Autodesk Fusion 360 part; units mm, degrees
(part 5 of 7)
  line L374 (70.3431, -42.6334) -> (70.3628, -42.5576)
  line L375 (70.3628, -42.5576) -> (70.3811, -42.4808)
  line L376 (70.3811, -42.4808) -> (70.2693, -42.3959)
  line L377 (70.2693, -42.3959) -> (70.1562, -42.3126)
  line L378 (70.1562, -42.3126) -> (70.0419, -42.2311)
  line L379 (70.0419, -42.2311) -> (69.974, -42.2713)
  line L380 (69.974, -42.2713) -> (69.9075, -42.3127)
  line L381 (69.9075, -42.3127) -> (69.8424, -42.3551)
  line L382 (69.8424, -42.3551) -> (69.7789, -42.3987)
  line L383 (69.7789, -42.3987) -> (69.7169, -42.4435)
  line L384 (69.7169, -42.4435) -> (69.6565, -42.4895)
  line L385 (69.6565, -42.4895) -> (69.5979, -42.5367)
  line L386 (69.5979, -42.5367) -> (69.5413, -42.5853)
  line L387 (69.5413, -42.5853) -> (69.4867, -42.6354)
  line L388 (69.4867, -42.6354) -> (69.4346, -42.6871)
  line L389 (69.4346, -42.6871) -> (69.3854, -42.7407)
  line L390 (69.3854, -42.7407) -> (69.3406, -42.7973)
  line L391 (69.3406, -42.7973) -> (69.0945, -43.1707)
  line L392 (69.0945, -43.1707) -> (68.9167, -43.0569)
  line L393 (68.9167, -43.0569) -> (68.7359, -42.9478)
  line L394 (68.7359, -42.9478) -> (68.5524, -42.8434)
  line L395 (68.5524, -42.8434) -> (68.3661, -42.744)
  line L396 (68.3661, -42.744) -> (68.5716, -42.3467)
  line L397 (68.5716, -42.3467) -> (68.599, -42.28)
  line L398 (68.599, -42.28) -> (68.6218, -42.2108)
  line L399 (68.6218, -42.2108) -> (68.6414, -42.1401)
  line L400 (68.6414, -42.1401) -> (68.6584, -42.068)
  line L401 (68.6584, -42.068) -> (68.6731, -41.9948)
  line L402 (68.6731, -41.9948) -> (68.6857, -41.9206)
  line L403 (68.6857, -41.9206) -> (68.6963, -41.8455)
  line L404 (68.6963, -41.8455) -> (68.705, -41.7695)
  line L405 (68.705, -41.7695) -> (68.712, -41.6928)
  line L406 (68.712, -41.6928) -> (68.7172, -41.6152)
  line L407 (68.7172, -41.6152) -> (68.7208, -41.537)
  line L408 (68.7208, -41.537) -> (68.7227, -41.4581)
  line L409 (68.7227, -41.4581) -> (68.5957, -41.3983)
  line L410 (68.5957, -41.3983) -> (68.4678, -41.3403)
  line L411 (68.4678, -41.3403) -> (68.339, -41.2843)
  line L412 (68.339, -41.2843) -> (68.2809, -41.3378)
  line L413 (68.2809, -41.3378) -> (68.2245, -41.3921)
  line L414 (68.2245, -41.3921) -> (68.1697, -41.4471)
  line L415 (68.1697, -41.4471) -> (68.1165, -41.503)
  line L416 (68.1165, -41.503) -> (68.0652, -41.5597)
  line L417 (68.0652, -41.5597) -> (68.0157, -41.6172)
  line L418 (68.0157, -41.6172) -> (67.9683, -41.6756)
  line L419 (67.9683, -41.6756) -> (67.923, -41.7349)
  line L420 (67.923, -41.7349) -> (67.88, -41.7952)
  line L421 (67.88, -41.7952) -> (67.8398, -41.8566)
  line L422 (67.8398, -41.8566) -> (67.8028, -41.9193)
  line L423 (67.8028, -41.9193) -> (67.7707, -41.984)
  line L424 (67.7707, -41.984) -> (67.6076, -42.4004)
  line L425 (67.6076, -42.4004) -> (67.41, -42.326)
  line L426 (67.41, -42.326) -> (67.2106, -42.2569)
  line L427 (67.2106, -42.2569) -> (67.0093, -42.193)
  line L428 (67.0093, -42.193) -> (66.8065, -42.1344)
  line L429 (66.8065, -42.1344) -> (66.9248, -41.7032)
  line L430 (66.9248, -41.7032) -> (66.9378, -41.6322)
  line L431 (66.9378, -41.6322) -> (66.9457, -41.5598)
  line L432 (66.9457, -41.5598) -> (66.9502, -41.4865)
  line L433 (66.9502, -41.4865) -> (66.9518, -41.4125)
  line L434 (66.9518, -41.4125) -> (66.951, -41.3378)
  line L435 (66.951, -41.3378) -> (66.9479, -41.2627)
  line L436 (66.9479, -41.2627) -> (66.9426, -41.187)
  line L437 (66.9426, -41.187) -> (66.9354, -41.1108)
  line L438 (66.9354, -41.1108) -> (66.9262, -41.0343)
  line L439 (66.9262, -41.0343) -> (66.9152, -40.9574)
  line L440 (66.9152, -40.9574) -> (66.9024, -40.8801)
  line L441 (66.9024, -40.8801) -> (66.8879, -40.8025)
  line L442 (66.8879, -40.8025) -> (66.7512, -40.7704)
  line L443 (66.7512, -40.7704) -> (66.614, -40.7403)
  line L444 (66.614, -40.7403) -> (66.4764, -40.7123)
  line L445 (66.4764, -40.7123) -> (66.4308, -40.7767)
  line L446 (66.4308, -40.7767) -> (66.3868, -40.8415)
  line L447 (66.3868, -40.8415) -> (66.3447, -40.9068)
  line L448 (66.3447, -40.9068) -> (66.3043, -40.9725)
  line L449 (66.3043, -40.9725) -> (66.2659, -41.0386)
  line L450 (66.2659, -41.0386) -> (66.2295, -41.1051)
  line L451 (66.2295, -41.1051) -> (66.1952, -41.1721)
  line L452 (66.1952, -41.1721) -> (66.1632, -41.2396)
  line L453 (66.1632, -41.2396) -> (66.1337, -41.3075)
  line L454 (66.1337, -41.3075) -> (66.1071, -41.3759)
  line L455 (66.1071, -41.3759) -> (66.084, -41.4449)
  line L456 (66.084, -41.4449) -> (66.066, -41.5149)
  line L457 (66.066, -41.5149) -> (65.9931, -41.9561)
  line L458 (65.9931, -41.9561) -> (65.7844, -41.9244)
  line L459 (65.7844, -41.9244) -> (65.5749, -41.8982)
  line L460 (65.5749, -41.8982) -> (65.3648, -41.8776)
  line L461 (65.3648, -41.8776) -> (65.1542, -41.8625)
  line L462 (65.1542, -41.8625) -> (65.1803, -41.416)
  line L463 (65.1803, -41.416) -> (65.1782, -41.3439)
  line L464 (65.1782, -41.3439) -> (65.1709, -41.2714)
  line L465 (65.1709, -41.2714) -> (65.16, -41.1988)
  line L466 (65.16, -41.1988) -> (65.1462, -41.1261)
  line L467 (65.1462, -41.1261) -> (65.1299, -41.0533)
  line L468 (65.1299, -41.0533) -> (65.1112, -40.9804)
  line L469 (65.1112, -40.9804) -> (65.0903, -40.9074)
  line L470 (65.0903, -40.9074) -> (65.0674, -40.8345)
  line L471 (65.0674, -40.8345) -> (65.0425, -40.7615)
  line L472 (65.0425, -40.7615) -> (65.0158, -40.6885)
  line L473 (65.0158, -40.6885) -> (64.9872, -40.6156)
  line L474 (64.9872, -40.6156) -> (64.9569, -40.5428)
  line L475 (64.9569, -40.5428) -> (64.8165, -40.5397)
  line L476 (64.8165, -40.5397) -> (64.6761, -40.5388)
  line L477 (64.6761, -40.5388) -> (64.5356, -40.5401)
  line L478 (64.5356, -40.5401) -> (64.5044, -40.6125)
  line L479 (64.5044, -40.6125) -> (64.4749, -40.6851)
  line L480 (64.4749, -40.6851) -> (64.4472, -40.7577)
  line L481 (64.4472, -40.7577) -> (64.4214, -40.8303)
  line L482 (64.4214, -40.8303) -> (64.3975, -40.903)
  line L483 (64.3975, -40.903) -> (64.3758, -40.9757)
  line L484 (64.3758, -40.9757) -> (64.3561, -41.0483)
  line L485 (64.3561, -41.0483) -> (64.3389, -41.1209)
  line L486 (64.3389, -41.1209) -> (64.3242, -41.1935)
  line L487 (64.3242, -41.1935) -> (64.3124, -41.2659)
  line L488 (64.3124, -41.2659) -> (64.3041, -41.3383)
  line L489 (64.3041, -41.3383) -> (64.3011, -41.4104)
  line L490 (64.3011, -41.4104) -> (64.3215, -41.8572)
  line L491 (64.3215, -41.8572) -> (64.1107, -41.8696)
  line L492 (64.1107, -41.8696) -> (63.9004, -41.8875)
  line L493 (63.9004, -41.8875) -> (63.6905, -41.911)
  line L494 (63.6905, -41.911) -> (63.4814, -41.94)
  line L495 (63.4814, -41.94) -> (63.4141, -41.4979)
  line L496 (63.4141, -41.4979) -> (63.3971, -41.4277)
  line L497 (63.3971, -41.4277) -> (63.3749, -41.3584)
  line L498 (63.3749, -41.3584) -> (63.3491, -41.2897)
  line L499 (63.3491, -41.2897) -> (63.3205, -41.2214)
  line L500 (63.3205, -41.2214) -> (63.2894, -41.1535)
  line L501 (63.2894, -41.1535) -> (63.256, -41.0861)
  line L502 (63.256, -41.0861) -> (63.2204, -41.0191)
  line L503 (63.2204, -41.0191) -> (63.1828, -40.9525)
  line L504 (63.1828, -40.9525) -> (63.1433, -40.8863)
  line L505 (63.1433, -40.8863) -> (63.102, -40.8205)
  line L506 (63.102, -40.8205) -> (63.0589, -40.7551)
  line L507 (63.0589, -40.7551) -> (63.0141, -40.6901)
  line L508 (63.0141, -40.6901) -> (62.8761, -40.7164)
  line L509 (62.8761, -40.7164) -> (62.7386, -40.7447)
  line L510 (62.7386, -40.7447) -> (62.6015, -40.7751)
  line L511 (62.6015, -40.7751) -> (62.5859, -40.8525)
  line L512 (62.5859, -40.8525) -> (62.5722, -40.9296)
  line L513 (62.5722, -40.9296) -> (62.5602, -41.0063)
  line L514 (62.5602, -41.0063) -> (62.5501, -41.0827)
  line L515 (62.5501, -41.0827) -> (62.5418, -41.1588)
  line L516 (62.5418, -41.1588) -> (62.5356, -41.2344)
  line L517 (62.5356, -41.2344) -> (62.5315, -41.3095)
  line L518 (62.5315, -41.3095) -> (62.5297, -41.3842)
  line L519 (62.5297, -41.3842) -> (62.5304, -41.4582)
  line L520 (62.5304, -41.4582) -> (62.534, -41.5315)
  line L521 (62.534, -41.5315) -> (62.5409, -41.604)
  line L522 (62.5409, -41.604) -> (62.553, -41.6752)
  line L523 (62.553, -41.6752) -> (62.6658, -42.1079)
  line L524 (62.6658, -42.1079) -> (62.4622, -42.1639)
  line L525 (62.4622, -42.1639) -> (62.2602, -42.2252)
  line L526 (62.2602, -42.2252) -> (62.0599, -42.2918)
  line L527 (62.0599, -42.2918) -> (61.8613, -42.3636)
  line L528 (61.8613, -42.3636) -> (61.7036, -41.9451)
  line L529 (61.7036, -41.9451) -> (61.6724, -41.8801)
  line L530 (61.6724, -41.8801) -> (61.6362, -41.8169)
  line L531 (61.6362, -41.8169) -> (61.5967, -41.755)
  line L532 (61.5967, -41.755) -> (61.5546, -41.6941)
  line L533 (61.5546, -41.6941) -> (61.51, -41.6342)
  line L534 (61.51, -41.6342) -> (61.4633, -41.5752)
  line L535 (61.4633, -41.5752) -> (61.4146, -41.5171)
  line L536 (61.4146, -41.5171) -> (61.3639, -41.4598)
  line L537 (61.3639, -41.4598) -> (61.3115, -41.4032)
  line L538 (61.3115, -41.4032) -> (61.2574, -41.3474)
  line L539 (61.2574, -41.3474) -> (61.2017, -41.2925)
  line L540 (61.2017, -41.2925) -> (61.1443, -41.2382)
  line L541 (61.1443, -41.2382) -> (61.0148, -41.2926)
  line L542 (61.0148, -41.2926) -> (60.8862, -41.3489)
  line L543 (60.8862, -41.3489) -> (60.7584, -41.4071)
  line L544 (60.7584, -41.4071) -> (60.7593, -41.486)
  line L545 (60.7593, -41.486) -> (60.7619, -41.5643)
  line L546 (60.7619, -41.5643) -> (60.7661, -41.6419)
  line L547 (60.7661, -41.6419) -> (60.7721, -41.7187)
  line L548 (60.7721, -41.7187) -> (60.7799, -41.7948)
  line L549 (60.7799, -41.7948) -> (60.7895, -41.8701)
  line L550 (60.7895, -41.8701) -> (60.8011, -41.9444)
  line L551 (60.8011, -41.9444) -> (60.8149, -42.0178)
  line L552 (60.8149, -42.0178) -> (60.831, -42.0901)
  line L553 (60.831, -42.0901) -> (60.8497, -42.1611)
  line L554 (60.8497, -42.1611) -> (60.8715, -42.2305)
  line L555 (60.8715, -42.2305) -> (60.8981, -42.2976)
  line L556 (60.8981, -42.2976) -> (61.0985, -42.6974)
  line L557 (61.0985, -42.6974) -> (60.911, -42.7945)
  line L558 (60.911, -42.7945) -> (60.7261, -42.8965)
  line L559 (60.7261, -42.8965) -> (60.544, -43.0033)
  line L560 (60.544, -43.0033) -> (60.3647, -43.1148)
  line L561 (60.3647, -43.1148) -> (60.1234, -42.7383)
  line L562 (60.1234, -42.7383) -> (60.0794, -42.6811)
  line L563 (60.0794, -42.6811) -> (60.0308, -42.6268)
  line L564 (60.0308, -42.6268) -> (59.9794, -42.5745)
  line L565 (59.9794, -42.5745) -> (59.9255, -42.5237)
  line L566 (59.9255, -42.5237) -> (59.8694, -42.4744)
  line L567 (59.8694, -42.4744) -> (59.8115, -42.4264)
  line L568 (59.8115, -42.4264) -> (59.7517, -42.3797)
  line L569 (59.7517, -42.3797) -> (59.6903, -42.3341)
  line L570 (59.6903, -42.3341) -> (59.6273, -42.2897)
  line L571 (59.6273, -42.2897) -> (59.5628, -42.2464)
  line L572 (59.5628, -42.2464) -> (59.4968, -42.2042)
  line L573 (59.4968, -42.2042) -> (59.4294, -42.1631)
  line L574 (59.4294, -42.1631) -> (59.3141, -42.2432)
  line L575 (59.3141, -42.2432) -> (59.1999, -42.325)
  line L576 (59.1999, -42.325) -> (59.087, -42.4085)
  line L577 (59.087, -42.4085) -> (59.1043, -42.4855)
  line L578 (59.1043, -42.4855) -> (59.1231, -42.5615)
  line L579 (59.1231, -42.5615) -> (59.1434, -42.6365)
  line L580 (59.1434, -42.6365) -> (59.1652, -42.7105)
  line L581 (59.1652, -42.7105) -> (59.1886, -42.7833)
  line L582 (59.1886, -42.7833) -> (59.2137, -42.8549)
  line L583 (59.2137, -42.8549) -> (59.2405, -42.9252)
  line L584 (59.2405, -42.9252) -> (59.2693, -42.9941)
  line L585 (59.2693, -42.9941) -> (59.3, -43.0614)
  line L586 (59.3, -43.0614) -> (59.3331, -43.127)
  line L587 (59.3331, -43.127) -> (59.3689, -43.1904)
  line L588 (59.3689, -43.1904) -> (59.4088, -43.2505)
  line L589 (59.4088, -43.2505) -> (59.6879, -43.5999)
  line L590 (59.6879, -43.5999) -> (59.5247, -43.7339)
  line L591 (59.5247, -43.7339) -> (59.3651, -43.872)
  line L592 (59.3651, -43.872) -> (59.2092, -44.0144)
  line L593 (59.2092, -44.0144) -> (59.057, -44.1608)
  line L594 (59.057, -44.1608) -> (58.7427, -43.8426)
  line L595 (58.7427, -43.8426) -> (58.6877, -43.7959)
  line L596 (58.6877, -43.7959) -> (58.629, -43.7529)
  line L597 (58.629, -43.7529) -> (58.5677, -43.7124)
  line L598 (58.5677, -43.7124) -> (58.5045, -43.6739)
  line L599 (58.5045, -43.6739) -> (58.4394, -43.6373)
  line L600 (58.4394, -43.6373) -> (58.3727, -43.6024)
  line L601 (58.3727, -43.6024) -> (58.3045, -43.5691)
  line L602 (58.3045, -43.5691) -> (58.235, -43.5373)
  line L603 (58.235, -43.5373) -> (58.1641, -43.507)
  line L604 (58.1641, -43.507) -> (58.092, -43.4781)
  line L605 (58.092, -43.4781) -> (58.0187, -43.4505)
  line L606 (58.0187, -43.4505) -> (57.9443, -43.4243)
  line L607 (57.9443, -43.4243) -> (57.8481, -43.5266)
  line L608 (57.8481, -43.5266) -> (57.7534, -43.6304)
  line L609 (57.7534, -43.6304) -> (57.6604, -43.7355)
  line L610 (57.6604, -43.7355) -> (57.6933, -43.8072)
  line L611 (57.6933, -43.8072) -> (57.7275, -43.8777)
  line L612 (57.7275, -43.8777) -> (57.7629, -43.9469)
  line L613 (57.7629, -43.9469) -> (57.7996, -44.0147)
  line L614 (57.7996, -44.0147) -> (57.8377, -44.081)
  line L615 (57.8377, -44.081) -> (57.8771, -44.1458)
  line L616 (57.8771, -44.1458) -> (57.918, -44.209)
  line L617 (57.918, -44.209) -> (57.9604, -44.2704)
  line L618 (57.9604, -44.2704) -> (58.0045, -44.3299)
  line L619 (58.0045, -44.3299) -> (58.0504, -44.3872)
  line L620 (58.0504, -44.3872) -> (58.0986, -44.4417)
  line L621 (58.0986, -44.4417) -> (58.1502, -44.4922)
  line L622 (58.1502, -44.4922) -> (58.4959, -44.776)
  line L623 (58.4959, -44.776) -> (58.3641, -44.9409)
  line L624 (58.3641, -44.9409) -> (58.2367, -45.1093)
  line L625 (58.2367, -45.1093) -> (58.1137, -45.2809)
  line L626 (58.1137, -45.2809) -> (57.9953, -45.4557)
  line L627 (57.9953, -45.4557) -> (57.6217, -45.2099)
  line L628 (57.6217, -45.2099) -> (57.5582, -45.1756)
  line L629 (57.5582, -45.1756) -> (57.4918, -45.1457)
  line L630 (57.4918, -45.1457) -> (57.4235, -45.1189)
  line L631 (57.4235, -45.1189) -> (57.3536, -45.0944)
  line L632 (57.3536, -45.0944) -> (57.2824, -45.0721)
  line L633 (57.2824, -45.0721) -> (57.2099, -45.0519)
  line L634 (57.2099, -45.0519) -> (57.1363, -45.0335)
  line L635 (57.1363, -45.0335) -> (57.0617, -45.0168)
  line L636 (57.0617, -45.0168) -> (56.986, -45.0019)
  line L637 (56.986, -45.0019) -> (56.9095, -44.9886)
  line L638 (56.9095, -44.9886) -> (56.832, -44.9769)
  line L639 (56.832, -44.9769) -> (56.7538, -44.9667)
  line L640 (56.7538, -44.9667) -> (56.681, -45.0868)
  line L641 (56.681, -45.0868) -> (56.61, -45.2079)
  line L642 (56.61, -45.2079) -> (56.5408, -45.3302)
  line L643 (56.5408, -45.3302) -> (56.5879, -45.3935)
  line L644 (56.5879, -45.3935) -> (56.636, -45.4553)
  line L645 (56.636, -45.4553) -> (56.6851, -45.5156)
  line L646 (56.6851, -45.5156) -> (56.7351, -45.5742)
  line L647 (56.7351, -45.5742) -> (56.7861, -45.6312)
  line L648 (56.7861, -45.6312) -> (56.8381, -45.6864)
  line L649 (56.8381, -45.6864) -> (56.8912, -45.7397)
  line L650 (56.8912, -45.7397) -> (56.9455, -45.791)
  line L651 (56.9455, -45.791) -> (57.001, -45.84)
  line L652 (57.001, -45.84) -> (57.0578, -45.8865)
  line L653 (57.0578, -45.8865) -> (57.1163, -45.9298)
  line L654 (57.1163, -45.9298) -> (57.1773, -45.9685)
  line L655 (57.1773, -45.9685) -> (57.5744, -46.1742)
  line L656 (57.5744, -46.1742) -> (57.4797, -46.3629)
  line L657 (57.4797, -46.3629) -> (57.3901, -46.5541)
  line L658 (57.3901, -46.5541) -> (57.3055, -46.7475)
  line L659 (57.3055, -46.7475) -> (57.2261, -46.9431)
  line L660 (57.2261, -46.9431) -> (56.8096, -46.7803)
  line L661 (56.8096, -46.7803) -> (56.7403, -46.76)
  line L662 (56.7403, -46.76) -> (56.6691, -46.7446)
  line L663 (56.6691, -46.7446) -> (56.5967, -46.7325)
  line L664 (56.5967, -46.7325) -> (56.5233, -46.7231)
  line L665 (56.5233, -46.7231) -> (56.449, -46.7162)
  line L666 (56.449, -46.7162) -> (56.3739, -46.7114)
  line L667 (56.3739, -46.7114) -> (56.2981, -46.7087)
  line L668 (56.2981, -46.7087) -> (56.2216, -46.708)
  line L669 (56.2216, -46.708) -> (56.1445, -46.7091)
  line L670 (56.1445, -46.7091) -> (56.0668, -46.712)
  line L671 (56.0668, -46.712) -> (55.9887, -46.7166)
  line L672 (55.9887, -46.7166) -> (55.91, -46.7229)
  line L673 (55.91, -46.7229) -> (55.8637, -46.8555)
  line L674 (55.8637, -46.8555) -> (55.8195, -46.9888)
  line L675 (55.8195, -46.9888) -> (55.7773, -47.1227)
  line L676 (55.7773, -47.1227) -> (55.8365, -47.1749)
  line L677 (55.8365, -47.1749) -> (55.8964, -47.2253)
  line L678 (55.8964, -47.2253) -> (55.9569, -47.2741)
  line L679 (55.9569, -47.2741) -> (56.018, -47.3211)
  line L680 (56.018, -47.3211) -> (56.0797, -47.3662)
  line L681 (56.0797, -47.3662) -> (56.1421, -47.4094)
  line L682 (56.1421, -47.4094) -> (56.2052, -47.4505)
  line L683 (56.2052, -47.4505) -> (56.2689, -47.4894)
  line L684 (56.2689, -47.4894) -> (56.3334, -47.5258)
  line L685 (56.3334, -47.5258) -> (56.3986, -47.5594)
  line L686 (56.3986, -47.5594) -> (56.4649, -47.5896)
  line L687 (56.4649, -47.5896) -> (56.5325, -47.6147)
  line L688 (56.5325, -47.6147) -> (56.9637, -47.7334)
  line L689 (56.9637, -47.7334) -> (56.9104, -47.9377)
  line L690 (56.9104, -47.9377) -> (56.8625, -48.1433)
  line L691 (56.8625, -48.1433) -> (56.82, -48.3501)
  line L692 (56.82, -48.3501) -> (56.7829, -48.558)
  line L693 (56.7829, -48.558) -> (56.3416, -48.4853)
  line L694 (56.3416, -48.4853) -> (56.2697, -48.4798)
  line L695 (56.2697, -48.4798) -> (56.1969, -48.4796)
  line L696 (56.1969, -48.4796) -> (56.1235, -48.4828)
  line L697 (56.1235, -48.4828) -> (56.0497, -48.4889)
  line L698 (56.0497, -48.4889) -> (55.9756, -48.4975)
  line L699 (55.9756, -48.4975) -> (55.9011, -48.5085)
  line L700 (55.9011, -48.5085) -> (55.8264, -48.5216)
  line L701 (55.8264, -48.5216) -> (55.7515, -48.5368)
  line L702 (55.7515, -48.5368) -> (55.6763, -48.5539)
  line L703 (55.6763, -48.5539) -> (55.6009, -48.5729)
  line L704 (55.6009, -48.5729) -> (55.5254, -48.5937)
  line L705 (55.5254, -48.5937) -> (55.4498, -48.6162)
  line L706 (55.4498, -48.6162) -> (55.4321, -48.7555)
  line L707 (55.4321, -48.7555) -> (55.4165, -48.8951)
  line L708 (55.4165, -48.8951) -> (55.4031, -49.0349)
  line L709 (55.4031, -49.0349) -> (55.4719, -49.0735)
  line L710 (55.4719, -49.0735) -> (55.5409, -49.1105)
  line L711 (55.5409, -49.1105) -> (55.6103, -49.1456)
  line L712 (55.6103, -49.1456) -> (55.6798, -49.1788)
  line L713 (55.6798, -49.1788) -> (55.7496, -49.2101)
  line L714 (55.7496, -49.2101) -> (55.8196, -49.2394)
  line L715 (55.8196, -49.2394) -> (55.8898, -49.2665)
  line L716 (55.8898, -49.2665) -> (55.9602, -49.2913)
  line L717 (55.9602, -49.2913) -> (56.0308, -49.3135)
  line L718 (56.0308, -49.3135) -> (56.1017, -49.3328)
  line L719 (56.1017, -49.3328) -> (56.1727, -49.3486)
  line L720 (56.1727, -49.3486) -> (56.2441, -49.3591)
  line L721 (56.2441, -49.3591) -> (56.6906, -49.3855)
  line L722 (56.6906, -49.3855) -> (56.6809, -49.5964)
  line L723 (56.6809, -49.5964) -> (56.6768, -49.8075)
  line L724 (56.6768, -49.8075) -> (56.6782, -50.0186)
  line L725 (56.6782, -50.0186) -> (56.6852, -50.2297)
  line L726 (56.6852, -50.2297) -> (56.2384, -50.2504)
  line L727 (56.2384, -50.2504) -> (56.1669, -50.26)
  line L728 (56.1669, -50.26) -> (56.0956, -50.2748)
  line L729 (56.0956, -50.2748) -> (56.0245, -50.2932)
  line L730 (56.0245, -50.2932) -> (55.9536, -50.3145)
  line L731 (55.9536, -50.3145) -> (55.8829, -50.3384)
  line L732 (55.8829, -50.3384) -> (55.8124, -50.3646)
  line L733 (55.8124, -50.3646) -> (55.742, -50.393)
  line L734 (55.742, -50.393) -> (55.6718, -50.4234)
  line L735 (55.6718, -50.4234) -> (55.6019, -50.4558)
  line L736 (55.6019, -50.4558) -> (55.5321, -50.49)
  line L737 (55.5321, -50.49) -> (55.4626, -50.526)
  line L738 (55.4626, -50.526) -> (55.3933, -50.5638)
  line L739 (55.3933, -50.5638) -> (55.405, -50.7037)
  line L740 (55.405, -50.7037) -> (55.4187, -50.8435)
  line L741 (55.4187, -50.8435) -> (55.4346, -50.983)
  line L742 (55.4346, -50.983) -> (55.51, -51.0065)
  line L743 (55.51, -51.0065) -> (55.5852, -51.0283)
  line L744 (55.5852, -51.0283) -> (55.6603, -51.0482)
  line L745 (55.6603, -51.0482) -> (55.7352, -51.0663)
  line L746 (55.7352, -51.0663) -> (55.81, -51.0824)
  line L747 (55.81, -51.0824) -> (55.8846, -51.0965)
  line L748 (55.8846, -51.0965) -> (55.9589, -51.1084)
  line L749 (55.9589, -51.1084) -> (56.0329, -51.118)
  line L750 (56.0329, -51.118) -> (56.1066, -51.1251)
  line L751 (56.1066, -51.1251) -> (56.1799, -51.1292)
  line L752 (56.1799, -51.1292) -> (56.2527, -51.1299)
  line L753 (56.2527, -51.1299) -> (56.3247, -51.1253)
  line L754 (56.3247, -51.1253) -> (56.7669, -51.0583)
  line L755 (56.7669, -51.0583) -> (56.8013, -51.2667)
  line L756 (56.8013, -51.2667) -> (56.8411, -51.474)
  line L757 (56.8411, -51.474) -> (56.8864, -51.6802)
  line L758 (56.8864, -51.6802) -> (56.9371, -51.8851)
  line L759 (56.9371, -51.8851) -> (56.5044, -51.9983)
  line L760 (56.5044, -51.9983) -> (56.4365, -52.0225)
  line L761 (56.4365, -52.0225) -> (56.3699, -52.0519)
  line L762 (56.3699, -52.0519) -> (56.3042, -52.0847)
  line L763 (56.3042, -52.0847) -> (56.2392, -52.1203)
  line L764 (56.2392, -52.1203) -> (56.175, -52.1583)
  line L765 (56.175, -52.1583) -> (56.1114, -52.1986)
  line L766 (56.1114, -52.1986) -> (56.0485, -52.241)
  line L767 (56.0485, -52.241) -> (55.9862, -52.2853)
  line L768 (55.9862, -52.2853) -> (55.9245, -52.3315)
  line L769 (55.9245, -52.3315) -> (55.8634, -52.3795)
  line L770 (55.8634, -52.3795) -> (55.8029, -52.4292)
  line L771 (55.8029, -52.4292) -> (55.7429, -52.4806)
  line L772 (55.7429, -52.4806) -> (55.7835, -52.615)
  line L773 (55.7835, -52.615) -> (55.826, -52.7489)
  line L774 (55.826, -52.7489) -> (55.8705, -52.882)
  line L775 (55.8705, -52.882) -> (55.9491, -52.8894)
  line L776 (55.9491, -52.8894) -> (56.0272, -52.895)
  line L777 (56.0272, -52.895) -> (56.1048, -52.8989)
  line L778 (56.1048, -52.8989) -> (56.1819, -52.901)
  line L779 (56.1819, -52.901) -> (56.2584, -52.9012)
  line L780 (56.2584, -52.9012) -> (56.3342, -52.8995)
  line L781 (56.3342, -52.8995) -> (56.4094, -52.8957)
  line L782 (56.4094, -52.8957) -> (56.4838, -52.8897)
  line L783 (56.4838, -52.8897) -> (56.5573, -52.8813)
  line L784 (56.5573, -52.8813) -> (56.6299, -52.8701)
  line L785 (56.6299, -52.8701) -> (56.7013, -52.8556)
  line L786 (56.7013, -52.8556) -> (56.7708, -52.8362)
  line L787 (56.7708, -52.8362) -> (57.1894, -52.6787)
  line L788 (57.1894, -52.6787) -> (57.2663, -52.8753)
  line L789 (57.2663, -52.8753) -> (57.3484, -53.0699)
  line L790 (57.3484, -53.0699) -> (57.4355, -53.2621)
  line L791 (57.4355, -53.2621) -> (57.5278, -53.4521)
  line L792 (57.5278, -53.4521) -> (57.1281, -53.6527)
  line L793 (57.1281, -53.6527) -> (57.0666, -53.6906)
  line L794 (57.0666, -53.6906) -> (57.0076, -53.7331)
  line L795 (57.0076, -53.7331) -> (56.9501, -53.7788)
  line L796 (56.9501, -53.7788) -> (56.894, -53.8271)
  line L797 (56.894, -53.8271) -> (56.8391, -53.8777)
  line L798 (56.8391, -53.8777) -> (56.7853, -53.9303)
  line L799 (56.7853, -53.9303) -> (56.7326, -53.9849)
  line L800 (56.7326, -53.9849) -> (56.6808, -54.0412)
  line L801 (56.6808, -54.0412) -> (56.6301, -54.0992)
  line L802 (56.6301, -54.0992) -> (56.5803, -54.1589)
  line L803 (56.5803, -54.1589) -> (56.5314, -54.2201)
  line L804 (56.5314, -54.2201) -> (56.4835, -54.2828)
  line L805 (56.4835, -54.2828) -> (56.5511, -54.4059)
  line L806 (56.5511, -54.4059) -> (56.6205, -54.5279)
  line L807 (56.6205, -54.5279) -> (56.6918, -54.6489)
  line L808 (56.6918, -54.6489) -> (56.7702, -54.6398)
  line L809 (56.7702, -54.6398) -> (56.8477, -54.6291)
  line L810 (56.8477, -54.6291) -> (56.9244, -54.6167)
  line L811 (56.9244, -54.6167) -> (57.0003, -54.6028)
  line L812 (57.0003, -54.6028) -> (57.0751, -54.5871)
  line L813 (57.0751, -54.5871) -> (57.1489, -54.5696)
  line L814 (57.1489, -54.5696) -> (57.2217, -54.5503)
  line L815 (57.2217, -54.5503) -> (57.2932, -54.5289)
  line L816 (57.2932, -54.5289) -> (57.3634, -54.5054)
  line L817 (57.3634, -54.5054) -> (57.432, -54.4794)
  line L818 (57.432, -54.4794) -> (57.4988, -54.4504)
  line L819 (57.4988, -54.4504) -> (57.5628, -54.4169)
  line L820 (57.5628, -54.4169) -> (57.9395, -54.1759)
  line L821 (57.9395, -54.1759) -> (58.0556, -54.3522)
  line L822 (58.0556, -54.3522) -> (58.1763, -54.5254)
  line L823 (58.1763, -54.5254) -> (58.3016, -54.6953)
  line L824 (58.3016, -54.6953) -> (58.4313, -54.8619)
  line L825 (58.4313, -54.8619) -> (58.082, -55.1413)
  line L826 (58.082, -55.1413) -> (58.0298, -55.1911)
  line L827 (58.0298, -55.1911) -> (57.9809, -55.245)
  line L828 (57.9809, -55.245) -> (57.9342, -55.3017)
  line L829 (57.9342, -55.3017) -> (57.8893, -55.3606)
  line L830 (57.8893, -55.3606) -> (57.8462, -55.4215)
  line L831 (57.8462, -55.4215) -> (57.8045, -55.4841)
  line L832 (57.8045, -55.4841) -> (57.7642, -55.5485)
  line L833 (57.7642, -55.5485) -> (57.7253, -55.6143)
  line L834 (57.7253, -55.6143) -> (57.6878, -55.6816)
  line L835 (57.6878, -55.6816) -> (57.6514, -55.7503)
  line L836 (57.6514, -55.7503) -> (57.6164, -55.8203)
  line L837 (57.6164, -55.8203) -> (57.5825, -55.8916)
  line L838 (57.5825, -55.8916) -> (57.6742, -55.998)
  line L839 (57.6742, -55.998) -> (57.7675, -56.1029)
  line L840 (57.7675, -56.1029) -> (57.8624, -56.2065)
  line L841 (57.8624, -56.2065) -> (57.9372, -56.1812)
  line L842 (57.9372, -56.1812) -> (58.0108, -56.1546)
  line L843 (58.0108, -56.1546) -> (58.0833, -56.1266)
  line L844 (58.0833, -56.1266) -> (58.1545, -56.0972)
  line L845 (58.1545, -56.0972) -> (58.2245, -56.0663)
  line L846 (58.2245, -56.0663) -> (58.2931, -56.0338)
  line L847 (58.2931, -56.0338) -> (58.3602, -55.9998)
  line L848 (58.3602, -55.9998) -> (58.4257, -55.964)
  line L849 (58.4257, -55.964) -> (58.4895, -55.9264)
  line L850 (58.4895, -55.9264) -> (58.5512, -55.8867)
  line L851 (58.5512, -55.8867) -> (58.6105, -55.8444)
  line L852 (58.6105, -55.8444) -> (58.6661, -55.7984)
  line L853 (58.6661, -55.7984) -> (58.9845, -55.4843)
  line L854 (58.9845, -55.4843) -> (59.1347, -55.6327)
  line L855 (59.1347, -55.6327) -> (59.2888, -55.777)
  line L856 (59.2888, -55.777) -> (59.4467, -55.9172)
  line L857 (59.4467, -55.9172) -> (59.6082, -56.0532)
  line L858 (59.6082, -56.0532) -> (59.3246, -56.399)
  line L859 (59.3246, -56.399) -> (59.2839, -56.4586)
  line L860 (59.2839, -56.4586) -> (59.2473, -56.5215)
  line L861 (59.2473, -56.5215) -> (59.2134, -56.5867)
  line L862 (59.2134, -56.5867) -> (59.1818, -56.6536)
  line L863 (59.1818, -56.6536) -> (59.1522, -56.7221)
  line L864 (59.1522, -56.7221) -> (59.1244, -56.7921)
  line L865 (59.1244, -56.7921) -> (59.0984, -56.8634)
  line L866 (59.0984, -56.8634) -> (59.0741, -56.9359)
  line L867 (59.0741, -56.9359) -> (59.0513, -57.0095)
  line L868 (59.0513, -57.0095) -> (59.0301, -57.0843)
  line L869 (59.0301, -57.0843) -> (59.0103, -57.16)
  line L870 (59.0103, -57.16) -> (58.992, -57.2368)
  line L871 (58.992, -57.2368) -> (59.1039, -57.3218)
  line L872 (59.1039, -57.3218) -> (59.2169, -57.405)
  line L873 (59.2169, -57.405) -> (59.3313, -57.4866)
  line L874 (59.3313, -57.4866) -> (59.3992, -57.4463)
  line L875 (59.3992, -57.4463) -> (59.4657, -57.405)
  line L876 (59.4657, -57.405) -> (59.5307, -57.3625)
  line L877 (59.5307, -57.3625) -> (59.5943, -57.3189)
  line L878 (59.5943, -57.3189) -> (59.6563, -57.2742)
  line L879 (59.6563, -57.2742) -> (59.7167, -57.2282)
  line L880 (59.7167, -57.2282) -> (59.7752, -57.1809)
  line L881 (59.7752, -57.1809) -> (59.8319, -57.1323)
  line L882 (59.8319, -57.1323) -> (59.8864, -57.0823)
  line L883 (59.8864, -57.0823) -> (59.9386, -57.0306)
  line L884 (59.9386, -57.0306) -> (59.9878, -56.9769)
  line L885 (59.9878, -56.9769) -> (60.0326, -56.9204)
  line L886 (60.0326, -56.9204) -> (60.2787, -56.5469)
  line L887 (60.2787, -56.5469) -> (60.4565, -56.6608)
  line L888 (60.4565, -56.6608) -> (60.6372, -56.7699)
  line L889 (60.6372, -56.7699) -> (60.8208, -56.8742)
  line L890 (60.8208, -56.8742) -> (61.007, -56.9737)
  line L891 (61.007, -56.9737) -> (60.8016, -57.3709)
  line L892 (60.8016, -57.3709) -> (60.7741, -57.4377)
  line L893 (60.7741, -57.4377) -> (60.7514, -57.5068)
  line L894 (60.7514, -57.5068) -> (60.7318, -57.5776)
  line L895 (60.7318, -57.5776) -> (60.7148, -57.6496)
  line L896 (60.7148, -57.6496) -> (60.7001, -57.7228)
  line L897 (60.7001, -57.7228) -> (60.6875, -57.797)
  line L898 (60.6875, -57.797) -> (60.6769, -57.8721)
  line L899 (60.6769, -57.8721) -> (60.6681, -57.9481)
  line L900 (60.6681, -57.9481) -> (60.6612, -58.0249)
  line L901 (60.6612, -58.0249) -> (60.6559, -58.1024)
  line L902 (60.6559, -58.1024) -> (60.6524, -58.1806)
  line L903 (60.6524, -58.1806) -> (60.6505, -58.2595)
  line L904 (60.6505, -58.2595) -> (60.7775, -58.3194)
  line L905 (60.7775, -58.3194) -> (60.9054, -58.3773)
  line L906 (60.9054, -58.3773) -> (61.0342, -58.4334)
  line L907 (61.0342, -58.4334) -> (61.0922, -58.3799)
  line L908 (61.0922, -58.3799) -> (61.1487, -58.3256)
  line L909 (61.1487, -58.3256) -> (61.2035, -58.2705)
  line L910 (61.2035, -58.2705) -> (61.2566, -58.2147)
  line L911 (61.2566, -58.2147) -> (61.308, -58.158)
  line L912 (61.308, -58.158) -> (61.3574, -58.1004)
  line L913 (61.3574, -58.1004) -> (61.4049, -58.0421)
  line L914 (61.4049, -58.0421) -> (61.4502, -57.9827)
  line L915 (61.4502, -57.9827) -> (61.4932, -57.9224)
  line L916 (61.4932, -57.9224) -> (61.5334, -57.861)
  line L917 (61.5334, -57.861) -> (61.5704, -57.7983)
  line L918 (61.5704, -57.7983) -> (61.6025, -57.7337)
  line L919 (61.6025, -57.7337) -> (61.7656, -57.3172)
  line L920 (61.7656, -57.3172) -> (61.9631, -57.3916)
  line L921 (61.9631, -57.3916) -> (62.1626, -57.4608)
  line L922 (62.1626, -57.4608) -> (62.3638, -57.5247)
  line L923 (62.3638, -57.5247) -> (62.5667, -57.5832)
  line L924 (62.5667, -57.5832) -> (62.4483, -58.0145)
  line L925 (62.4483, -58.0145) -> (62.4354, -58.0855)
  line L926 (62.4354, -58.0855) -> (62.4275, -58.1579)
  line L927 (62.4275, -58.1579) -> (62.423, -58.2312)
  line L928 (62.423, -58.2312) -> (62.4214, -58.3052)
  line L929 (62.4214, -58.3052) -> (62.4222, -58.3798)
  line L930 (62.4222, -58.3798) -> (62.4253, -58.455)
  line L931 (62.4253, -58.455) -> (62.4306, -58.5307)
  line L932 (62.4306, -58.5307) -> (62.4378, -58.6068)
  line L933 (62.4378, -58.6068) -> (62.447, -58.6834)
  line L934 (62.447, -58.6834) -> (62.458, -58.7603)
  line L935 (62.458, -58.7603) -> (62.4707, -58.8376)
  line L936 (62.4707, -58.8376) -> (62.4853, -58.9151)
  line L937 (62.4853, -58.9151) -> (62.622, -58.9473)
  line L938 (62.622, -58.9473) -> (62.7591, -58.9773)
  line L939 (62.7591, -58.9773) -> (62.8967, -59.0054)
  line L940 (62.8967, -59.0054) -> (62.9424, -58.941)
  line L941 (62.9424, -58.941) -> (62.9863, -58.8761)
  line L942 (62.9863, -58.8761) -> (63.0285, -58.8109)
  line L943 (63.0285, -58.8109) -> (63.0689, -58.7452)
  line L944 (63.0689, -58.7452) -> (63.1073, -58.6791)
  line L945 (63.1073, -58.6791) -> (63.1437, -58.6125)
  line L946 (63.1437, -58.6125) -> (63.178, -58.5455)
  line L947 (63.178, -58.5455) -> (63.21, -58.4781)
  line L948 (63.21, -58.4781) -> (63.2395, -58.4102)
  line L949 (63.2395, -58.4102) -> (63.2661, -58.3417)
  line L950 (63.2661, -58.3417) -> (63.2892, -58.2727)
  line L951 (63.2892, -58.2727) -> (63.3071, -58.2028)
  line L952 (63.3071, -58.2028) -> (63.3801, -57.7616)
  line L953 (63.3801, -57.7616) -> (63.5888, -57.7932)
  line L954 (63.5888, -57.7932) -> (63.7983, -57.8194)
  line L955 (63.7983, -57.8194) -> (64.0084, -57.8401)
  line L956 (64.0084, -57.8401) -> (64.219, -57.8552)
  line L957 (64.219, -57.8552) -> (64.1929, -58.3016)
  line L958 (64.1929, -58.3016) -> (64.195, -58.3738)
  line L959 (64.195, -58.3738) -> (64.2023, -58.4462)
  line L960 (64.2023, -58.4462) -> (64.2132, -58.5188)
  line L961 (64.2132, -58.5188) -> (64.227, -58.5916)
  line L962 (64.227, -58.5916) -> (64.2433, -58.6644)
  line L963 (64.2433, -58.6644) -> (64.262, -58.7373)
  line L964 (64.262, -58.7373) -> (64.2828, -58.8102)
  line L965 (64.2828, -58.8102) -> (64.3058, -58.8832)
  line L966 (64.3058, -58.8832) -> (64.3306, -58.9562)
  line L967 (64.3306, -58.9562) -> (64.3574, -59.0291)
  line L968 (64.3574, -59.0291) -> (64.3859, -59.102)
  line L969 (64.3859, -59.102) -> (64.4163, -59.1749)
  line L970 (64.4163, -59.1749) -> (64.5567, -59.1779)
  line L971 (64.5567, -59.1779) -> (64.6971, -59.1788)
  line L972 (64.6971, -59.1788) -> (64.8375, -59.1776)
  line L973 (64.8375, -59.1776) -> (64.8688, -59.1051)
  line L974 (64.8688, -59.1051) -> (64.8983, -59.0326)
  line L975 (64.8983, -59.0326) -> (64.926, -58.96)
  line L976 (64.926, -58.96) -> (64.9518, -58.8873)
  line L977 (64.9518, -58.8873) -> (64.9756, -58.8147)
  line L978 (64.9756, -58.8147) -> (64.9974, -58.742)
  line L979 (64.9974, -58.742) -> (65.017, -58.6694)
  line L980 (65.017, -58.6694) -> (65.0343, -58.5967)
  line L981 (65.0343, -58.5967) -> (65.049, -58.5242)
  line L982 (65.049, -58.5242) -> (65.0608, -58.4517)
  line L983 (65.0608, -58.4517) -> (65.0691, -58.3794)
  line L984 (65.0691, -58.3794) -> (65.0721, -58.3073)
  line L985 (65.0721, -58.3073) -> (65.0517, -57.8605)
  line L986 (65.0517, -57.8605) -> (65.2625, -57.8481)
  line L987 (65.2625, -57.8481) -> (65.4728, -57.8302)
  line L988 (65.4728, -57.8302) -> (65.6826, -57.8067)
  line L989 (65.6826, -57.8067) -> (65.8918, -57.7776)
extrude "Extrude1'''" add sketch "Sketch1 (4)" along normal blind 1.8 separate body makes body 6 in component "CT idler 3"
ref_plane "WorkPlane2" through (0, 0, 43) normal (0, 0, 1) x (1, 0, 0) in component "CT idler 3"